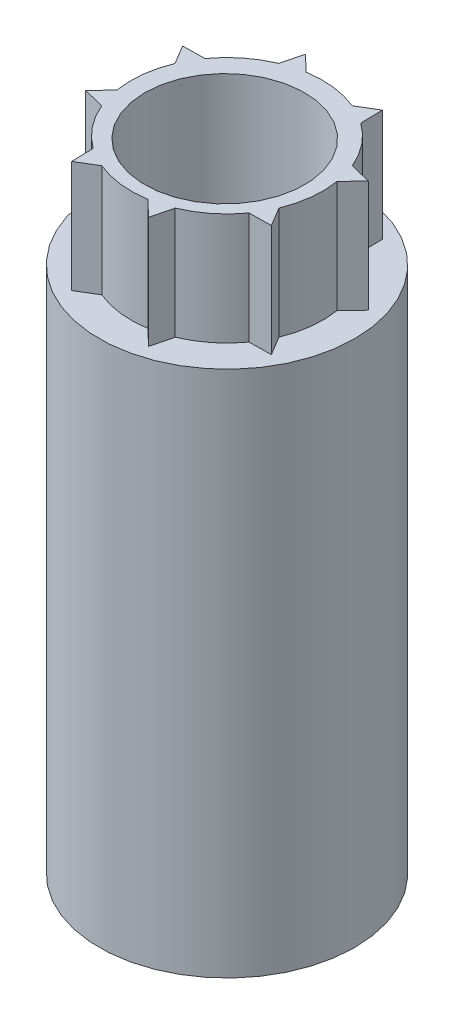
# Autodesk Inventor part: handle_base2
Saved by Autodesk Inventor 2021 (Build 250183000, 183)
## iProperties
Created: 2021-07-03
Part Number: handle_base2
Material: Generic
Document SubType Name: Modeling
Designer: teh18
Density: 1 g/cm^3
Appearance: Default
Author: teh18
Autodesk Inventor part; units mm, degrees
ref_plane "YZ Plane" through (0, 0, 0) normal (1, 0, 0) x (0, 1, 0)
ref_plane "XZ Plane" through (0, 0, 0) normal (0, 1, 0) x (-1, 0, 0)
ref_plane "XY Plane" through (0, 0, 0) normal (0, 0, 1) x (1, 0, 0)
sketch "Sketch4" plane through (0, 0, 0) normal (0, 1, 0) x (-1, 0, 0)
  point P0 (0, 0)
sketch "Sketch5" plane through (0, 0, 0) normal (0, 1, 0) x (-1, 0, 0)
  circle A0 centre (0, 0) radius 29.25 projected
  line L0 (-3.4978, -4.875) -> (-3.4751, -6.2541) projected
  line L1 (-3.4751, -6.2541) -> (-2.2921, -5.5449) projected
  arc A1 (-2.2921, -5.5449) -> (0.9738, -5.9204) centre (0, 0) ccw projected
  line L2 (0.9738, -5.9204) -> (1.965, -6.8796) projected
  line L3 (1.965, -6.8796) -> (2.3001, -5.5416) projected
  arc A2 (2.3001, -5.5416) -> (4.875, -3.4978) centre (0, 0) ccw projected
  line L4 (4.875, -3.4978) -> (6.2541, -3.4751) projected
  line L5 (6.2541, -3.4751) -> (5.5449, -2.2921) projected
  arc A3 (5.5449, -2.2921) -> (5.9204, 0.9738) centre (0, 0) ccw projected
  line L6 (5.9204, 0.9738) -> (6.8796, 1.965) projected
  line L7 (6.8796, 1.965) -> (5.5416, 2.3001) projected
  arc A4 (5.5416, 2.3001) -> (3.4978, 4.875) centre (0, 0) ccw projected
  line L8 (3.4978, 4.875) -> (3.4751, 6.2541) projected
  line L9 (3.4751, 6.2541) -> (2.2921, 5.5449) projected
  arc A5 (2.2921, 5.5449) -> (-0.9738, 5.9204) centre (0, 0) ccw projected
  line L10 (-0.9738, 5.9204) -> (-1.965, 6.8796) projected
  line L11 (-1.965, 6.8796) -> (-2.3001, 5.5416) projected
  arc A6 (-2.3001, 5.5416) -> (-4.875, 3.4978) centre (0, 0) ccw projected
  line L12 (-4.875, 3.4978) -> (-6.2541, 3.4751) projected
  line L13 (-6.2541, 3.4751) -> (-5.5449, 2.2921) projected
  arc A7 (-5.5449, 2.2921) -> (-5.9204, -0.9738) centre (0, 0) ccw projected
  line L14 (-5.9204, -0.9738) -> (-6.8796, -1.965) projected
  line L15 (-6.8796, -1.965) -> (-5.5416, -2.3001) projected
  arc A8 (-5.5416, -2.3001) -> (-3.4978, -4.875) centre (0, 0) ccw projected
  circle A9 centre (-0.0908, 0.2329) radius 5 projected
  point P0 (0, 0)
extrude "Extrusion4" add sketch "Sketch5" along normal blind 2 and the other way blind 5 contours A8 L15 L14 A7 L13 L12 A6 L11 L10 A5 L9 L8 A4 L7 L6 A3 L5 L4 A2 L3 L2 A1 L1 L0
sketch "Sketch6" plane through (0, -5, 0) normal (0, -1, 0) x (1, 0, 0)
  line L0 (2.2921, -5.5449) -> (3.4751, -6.2541) projected
  line L1 (3.4751, -6.2541) -> (3.4978, -4.875) projected
  arc A0 (3.4978, -4.875) -> (5.5416, -2.3001) centre (0, 0) ccw projected
  line L2 (5.5416, -2.3001) -> (6.8796, -1.965) projected
  line L3 (6.8796, -1.965) -> (5.9204, -0.9738) projected
  arc A1 (5.9204, -0.9738) -> (5.5449, 2.2921) centre (0, 0) ccw projected
  line L4 (5.5449, 2.2921) -> (6.2541, 3.4751) projected
  line L5 (6.2541, 3.4751) -> (4.875, 3.4978) projected
  arc A2 (4.875, 3.4978) -> (2.3001, 5.5416) centre (0, 0) ccw projected
  line L6 (2.3001, 5.5416) -> (1.965, 6.8796) projected
  line L7 (1.965, 6.8796) -> (0.9738, 5.9204) projected
  arc A3 (0.9738, 5.9204) -> (-2.2921, 5.5449) centre (0, 0) ccw projected
  line L8 (-2.2921, 5.5449) -> (-3.4751, 6.2541) projected
  line L9 (-3.4751, 6.2541) -> (-3.4978, 4.875) projected
  arc A4 (-3.4978, 4.875) -> (-5.5416, 2.3001) centre (0, 0) ccw projected
  line L10 (-5.5416, 2.3001) -> (-6.8796, 1.965) projected
  line L11 (-6.8796, 1.965) -> (-5.9204, 0.9738) projected
  arc A5 (-5.9204, 0.9738) -> (-5.5449, -2.2921) centre (0, 0) ccw projected
  line L12 (-5.5449, -2.2921) -> (-6.2541, -3.4751) projected
  line L13 (-6.2541, -3.4751) -> (-4.875, -3.4978) projected
  arc A6 (-4.875, -3.4978) -> (-2.3001, -5.5416) centre (0, 0) ccw projected
  line L14 (-2.3001, -5.5416) -> (-1.965, -6.8796) projected
  line L15 (-1.965, -6.8796) -> (-0.9738, -5.9204) projected
  arc A7 (-0.9738, -5.9204) -> (2.2921, -5.5449) centre (0, 0) ccw projected
  circle A8 centre (0.0908, 0.2329) radius 5 projected
  circle A9 centre (0, 0) radius 6
  circle A10 centre (0, 0) radius 8
  point P0 (0, 0)
  point P1 (-5.5416, 2.3001)
  point P2 (-5.5449, -2.2921)
  point P3 (-2.3001, -5.5416)
  point P4 (5.5416, -2.3001)
  point P5 (5.5449, 2.2921)
  point P6 (2.3001, 5.5416)
  point P7 (-2.2921, 5.5449)
  dimension "d15" = 2
  constraints: 2 centre point, 1 coincident, 1 concentric
  measures "d15" radial gap between concentric circles of A9 A10
extrude "Extrusion5" add sketch "Sketch6" along normal blind 33 contours A9 L1 L0 | A7 A9 A6 A5 A4 A3 A2 A1 A0 | L15 L14 A9 | A9 L3 L2 | L13 L12 A9 | L11 L10 A9 | A9 L5 L4 | L9 L8 A9 | A9 L7 L6 | A10
sketch "Sketch8" plane through (0, -38, 0) normal (0, -1, 0) x (1, 0, 0)
  circle A0 centre (0, 0) radius 8 projected
  circle A1 centre (0, 0) radius 6.1
  point P0 (0, 0)
  dimension "d19" = 12.2
  constraints: 1 centre point, 1 coincident
  measures "d19" diameter of A1
extrude "Extrusion7" cut sketch "Sketch8" against normal blind 10 contours A1
body "Solid2"
